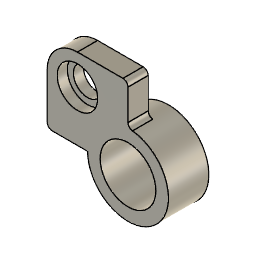
lesson 1 (Autodesk Fusion 360 design; units mm, degrees)
part number: 2025-10-31-10-40-48-589
Autodesk Fusion 360 part; units mm, degrees
note: some values were not read from the file. Set by a fixed rule: which sketch regions a step uses; the direction of a hole.
sketch "Sketch1" plane through (0, 0, 0) normal (0, 1, 0) x (1, 0, 0)
  circle A0 centre (0, 0) radius 0.6875
  circle A1 centre (0, 0) radius 1
  line L0 (0, 0) -> (-2, 0)
  line L1 (-2, 0) -> (-2, -2)
  line L2 (-2, -2) -> (0, -2)
  line L3 (0, -2) -> (0, 0)
  point P0 (-1.25, -1.25)
  dimension "d1" = 1.375
  dimension "d2" = 2
  dimension "d3" = 2
  dimension "d4" = 2
  dimension "d5" = 1.25
  dimension "d6" = 1.25
  constraint coincident A0.centre A1.centre
  constraint concentric A0 A1
  constraint horizontal L0
  constraint vertical L1
  constraint horizontal L2
  constraint vertical L3
  measures "d1" diameter of A0
  measures "d2" diameter of A1
  measures "d3" distance of A0.centre L0.end
  measures "d4" distance of A0.centre L2.end
  measures "d5" distance of L0 P0
  measures "d6" distance of L3 P0
extrude "Extrude1" add sketch "Sketch1" along normal blind 1 contours A0 A1 L0 L3 | A0 A1 L0 L3
extrude "Extrude2" add sketch "Sketch1" along normal blind 0.5 contours A1 L0 L1 L2 L3
hole "Hole1" at (-1.25, 0, 1.25) direction (0, 1, 0) diameter 0.7 end through all counterbore diameter 1 counterbore depth 0.25
fillet "Fillet1" radius 0.125 1 edges at (0, 0.25, 1)
fillet "Fillet2" radius 0.125 1 edges at (0, 0.25, 2)
fillet "Fillet3" radius 0.125 1 edges at (-2, 0.25, 0)
fillet "Fillet4" radius 0.75 1 edges at (-2, 0.25, 2)
